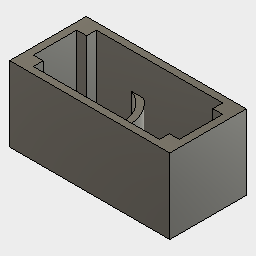
MG996R Body (Autodesk Fusion 360 design; units mm, degrees)
Autodesk Fusion 360 part; units mm, degrees
sketch "Base Sketch" plane through (0, 0, 0) normal (0, 1, 0) x (1, 0, 0)
  circle A0 centre (0, 0) radius 2.5 construction
  line L0 (-1.8028, 3) -> (1.8028, 3) construction
  line L1 (-1.8028, -3) -> (1.8028, -3) construction
  arc A1 (-1.8028, 3) -> (-1.8028, -3) centre (0, 0) ccw construction
  arc A2 (1.8028, -3) -> (1.8028, 3) centre (0, 0) ccw construction
  line L2 (-5, 5) -> (8, 5) construction
  line L3 (8, 5) -> (8, -5) construction
  line L4 (8, -5) -> (-5, -5) construction
  line L5 (-5, -5) -> (-5, 5) construction
  line L6 (8, 6) -> (-6, 6) construction
  line L7 (-6, 6) -> (-6, -6) construction
  line L8 (-6, -6) -> (8, -6) construction
  line L9 (8, -6) -> (8, 6) construction
  line L10 (8, 2.5) -> (6, 2.5) construction
  line L11 (6, 2.5) -> (6, 1.5) construction
  line L12 (6, 1.5) -> (8, 1.5) construction
  line L13 (8, 1.5) -> (8, 2.5) construction
  line L14 (8, -1.5) -> (6, -1.5) construction
  line L15 (6, -1.5) -> (6, -2.5) construction
  line L16 (6, -2.5) -> (8, -2.5) construction
  line L17 (8, -2.5) -> (8, -1.5) construction
  line L18 (-5, -6) -> (-1, -6) construction
  line L19 (-1, -6) -> (-1, -4) construction
  line L20 (-1, -4) -> (-5, -4) construction
  line L21 (-5, -4) -> (-5, -6) construction
  line L22 (2.5, 6) -> (6.5, 6) construction
  line L23 (6.5, 6) -> (6.5, 4) construction
  line L24 (6.5, 4) -> (2.5, 4) construction
  line L25 (2.5, 4) -> (2.5, 6) construction
  circle A3 centre (-20.5, 0) radius 8.5 construction
  circle A4 centre (-20.5, 0) radius 10 construction
  line L26 (8, 8) -> (-29, 8) construction
  line L27 (-29, 8) -> (-29, -8) construction
  line L28 (-29, -8) -> (8, -8) construction
  line L29 (8, -8) -> (8, 8) construction
  dimension "d1" = 5
  dimension "d2" = 7
  dimension "d3" = 6
  dimension "d4" = 3
  dimension "d5" = 10
  dimension "d6" = 5
  dimension "d7" = 5
  dimension "d8" = 13
  dimension "d9" = 1
  dimension "d10" = 1
  dimension "d11" = 1
  dimension "d12" = 2.5
  dimension "d13" = 2.5
  dimension "d14" = 1
  dimension "d15" = 2
  dimension "d16" = 4
  dimension "d17" = 2
  dimension "d18" = 4
  dimension "d19" = 2
  dimension "d20" = 7.5
  dimension "d21" = 17
  dimension "d22" = 1.5
  dimension "d23" = 4.5
  dimension "d24" = 37
  dimension "d25" = 16
  constraint coincident A0.centre A1.centre
  constraint horizontal L0
  constraint coincident A0.centre A1
  constraint parallel L0 L1
  constraint concentric A1 A2
  constraint horizontal L2
  constraint vertical L3
  constraint horizontal L4
  constraint vertical L5
  constraint horizontal L6
  constraint vertical L7
  constraint horizontal L8
  constraint vertical L9
  constraint collinear L3 L9
  constraint horizontal L10
  constraint vertical L11
  constraint horizontal L12
  constraint vertical L13
  constraint coincident L3 A0.centre
  constraint horizontal L14
  constraint vertical L15
  constraint horizontal L16
  constraint vertical L17
  constraint equal L10 L14
  constraint equal L11 L15
  constraint horizontal L18
  constraint vertical L19
  constraint horizontal L20
  constraint vertical L21
  constraint coincident L8 A0.centre
  constraint collinear L5 L21
  constraint horizontal L22
  constraint vertical L23
  constraint horizontal L24
  constraint vertical L25
  constraint coincident L6 A0.centre
  constraint horizontal A0.centre A1.centre
  constraint concentric A3 A4
  constraint coincident A4 A0.centre
  constraint horizontal L26
  constraint vertical L27
  constraint horizontal L28
  constraint vertical L29
  constraint collinear L3 L29
  constraint coincident L27 A0.centre
  constraint midpoint L27 A0.centre
  measures "d1" diameter of A0
  measures "d2" diameter of A1
  measures "d3" distance of L0 L1
  measures "d9" distance of L2 L6
  measures "d10" distance of L5 L7
  measures "d11" distance of L4 L8
  measures "d12" distance of L2 L10
  measures "d13" distance of L4 L16
  measures "d14" distance of A0.centre
  measures "d20" distance of L5 L25
  measures "d21" diameter of A3
  measures "d22" distance of A3 A4
sketch "Sketch2" plane through (0, 0, 0) normal (0, 1, 0) x (1, 0, 0)
  line L0 (8, 6) -> (-6, 6)
  line L1 (8, 5) -> (8, 6)
  line L2 (-6, 6) -> (-6, -6)
  line L3 (-6, -6) -> (8, -6)
  line L4 (8, -6) -> (8, -5)
  line L5 (8, -5) -> (-5, -5)
  line L6 (-5, -5) -> (-5, 5)
  line L7 (-5, 5) -> (8, 5)
extrude "Extrude1" add sketch "Sketch2" along normal blind 3.5 makes body 1
sketch "Sketch3" plane through (0, 3.5, 0) normal (0, 1, 0) x (-1, 0, 0)
  line L0 (5, -5) -> (-8, -5)
  line L1 (-8, -5) -> (-8, -6)
  line L2 (-8, -6) -> (6, -6)
  line L3 (6, -6) -> (6, 6)
  line L4 (6, 6) -> (-8, 6)
  line L5 (-8, 6) -> (-8, 5)
  line L6 (-8, 5) -> (5, 5)
  line L7 (5, 5) -> (5, -5)
  line L8 (-6.5, -5) -> (-2.5, -5)
  line L9 (-2.5, -5) -> (-2.5, -6)
  line L10 (-2.5, -6) -> (-6.5, -6)
  line L11 (-6.5, -6) -> (-6.5, -5)
  line L12 (-6.5, -6) -> (-6.5, -4)
  line L13 (5, 6) -> (1, 6)
  line L14 (1, 6) -> (1, 5)
  line L15 (1, 5) -> (5, 5)
  line L16 (5, 5) -> (5, 6)
  line L17 (1, 6) -> (1, 4)
  constraint horizontal L8
  constraint vertical L9
  constraint horizontal L10
  constraint vertical L11
  constraint midpoint origin L12
  constraint horizontal L13
  constraint vertical L14
  constraint horizontal L15
  constraint vertical L16
  constraint midpoint origin L17
extrude "Extrude2" add sketch "Sketch3" along normal blind 2.5 contours L0 L2 L8 L9 L10 L11 L12 | L4 L6 L13 L14 L15 L16 L17 bodies 1
sketch "Sketch4" plane through (0, 6, 0) normal (0, 1, 0) x (-1, 0, 0)
  line L0 (-2.5, -4) -> (-6.5, -4)
  line L1 (-6.5, -4) -> (-6.5, -6)
  line L2 (-6.5, -6) -> (-2.5, -6)
  line L3 (-2.5, -6) -> (-2.5, -4)
  line L4 (1, 4) -> (5, 4)
  line L5 (5, 4) -> (5, 6)
  line L6 (5, 6) -> (1, 6)
  line L7 (1, 6) -> (1, 4)
  constraint horizontal L0
  constraint vertical L1
  constraint horizontal L2
  constraint vertical L3
  constraint horizontal L4
  constraint vertical L5
  constraint horizontal L6
  constraint vertical L7
extrude "Extrude3" add sketch "Sketch4" along normal blind 1.5 bodies 1
sketch "Sketch5" plane through (0, 0, 0) normal (0, 1, 0) x (1, 0, 0)
  line L0 (8, 2.5) -> (6, 2.5)
  line L1 (6, 2.5) -> (6, 1.5)
  line L2 (6, 1.5) -> (8, 1.5)
  line L3 (8, 1.5) -> (8, 2.5)
  line L4 (6, -1.5) -> (8, -1.5)
  line L5 (8, -1.5) -> (8, -2.5)
  line L6 (8, -2.5) -> (6, -2.5)
  line L7 (6, -2.5) -> (6, -1.5)
  constraint horizontal L0
  constraint vertical L1
  constraint horizontal L2
  constraint vertical L3
  constraint horizontal L4
  constraint vertical L5
  constraint horizontal L6
  constraint vertical L7
extrude "Extrude4" add sketch "Sketch5" along normal blind 3.5 separate body makes body 2 at (6.6667, 2.3333, -2.5) makes body 3 at (6.6667, 2.3333, 2.5)
sketch "Sketch6" plane through (0, 0, 0) normal (0, 1, 0) x (1, 0, 0)
  circle A0 centre (0, 0) radius 2.5
  circle A1 centre (0, 0) radius 2.5
  arc A2 (1.8028, -3) -> (1.8028, 3) centre (0, 0) ccw
  line L0 (-1.8028, 3) -> (1.8028, 3)
  line L1 (-1.8028, -3) -> (1.8028, -3)
  arc A3 (1.8028, -3) -> (1.8028, 3) centre (0, 0) ccw
  arc A4 (-1.8028, 3) -> (-1.8028, -3) centre (0, 0) ccw
  constraint coincident A0.centre A1.centre
  constraint concentric A3 A4
extrude "Extrude5" add sketch "Sketch6" along normal blind 1 separate body makes body 4
sketch "Sketch7" plane through (0, 0, 0) normal (0, 1, 0) x (1, 0, 0)
  circle A0 centre (-20.5, 0) radius 8.5
  circle A1 centre (-20.5, 0) radius 8.5
  circle A2 centre (-20.5, 0) radius 10
  line L0 (-14.5, 8) -> (-17.6277, 8)
  line L1 (-14.5, -8) -> (-17.6277, -8)
  line L2 (-29, -8) -> (8, -8)
  line L3 (8, 8) -> (-29, 8)
  arc A3 (-17.6277, -8) -> (-17.6277, 8) centre (-20.5, 0) ccw
  arc A4 (-14.5, -8) -> (-14.5, 8) centre (-20.5, 0) ccw
  constraint coincident A2 origin
  constraint coincident A1 origin
  constraint parallel L0 L1
  constraint collinear L1 L2
  constraint collinear L0 L3
extrude "Extrude6" add sketch "Sketch7" along normal blind 10 separate body contours A0 A1 A2 L0 L1 L2 L3 A3 A4 makes body 5
sketch "Sketch8" plane through (0, 0, 0) normal (0, 1, 0) x (1, 0, 0)
  line L0 (-30.8, 9.7) -> (9.8, 9.7)
  line L1 (9.8, 9.7) -> (9.8, -9.7)
  line L2 (9.8, -9.7) -> (-30.8, -9.7)
  line L3 (-30.8, -9.7) -> (-30.8, 9.7)
  line L4 (8, -8) -> (8, 8)
  line L5 (-29, 8) -> (-29, -8)
  line L6 (8, 8) -> (-29, 8)
  line L7 (-29, -8) -> (8, -8)
  line L8 (-29, 8) -> (8, 8)
  line L9 (8, 8) -> (8, -8)
  line L10 (8, -8) -> (-29, -8)
  line L11 (-29, -8) -> (-29, 8)
  dimension "d38" = 1.8
  dimension "d39" = 1.8
  dimension "d40" = 1.7
  dimension "d41" = 1.7
  constraint horizontal L0
  constraint vertical L1
  constraint horizontal L2
  constraint vertical L3
  constraint horizontal L8
  constraint vertical L9
  constraint horizontal L10
  constraint vertical L11
  measures "d38" distance of L1 L4
  measures "d39" distance of L3 L5
  measures "d40" distance of L0 L6
  measures "d41" distance of L2 L7
extrude "Extrude7" add sketch "Sketch8" along normal blind 19 bodies 1 2 3 5
chamfer "Chamfer1" distance 1 angle 45 1 edges at (-3, 7.5, 4) on bodies 1
chamfer "Chamfer2" distance 1 angle 45 1 edges at (4.5, 7.5, -4) on bodies 1
sketch "Sketch9" plane through (0, 0, 0) normal (0, 1, 0) x (1, 0, 0)
  line L0 (-29, 8) -> (-26.5, 8)
  line L1 (-26.5, 8) -> (-26.5, 5.5)
  line L2 (-26.5, 5.5) -> (-29, 5.5)
  line L3 (-29, 5.5) -> (-29, 8)
  line L4 (-29, -8) -> (-26.5, -8)
  line L5 (-26.5, -8) -> (-26.5, -5.5)
  line L6 (-26.5, -5.5) -> (-29, -5.5)
  line L7 (-29, -5.5) -> (-29, -8)
  line L8 (8, 8) -> (5.5, 8)
  line L9 (5.5, 8) -> (5.5, 5.5)
  line L10 (5.5, 5.5) -> (8, 5.5)
  line L11 (8, 5.5) -> (8, 8)
  line L12 (8, -8) -> (5.5, -8)
  line L13 (5.5, -8) -> (5.5, -5.5)
  line L14 (5.5, -5.5) -> (8, -5.5)
  line L15 (8, -5.5) -> (8, -8)
  dimension "d46" = 2.5
  dimension "d47" = 2.5
  dimension "d48" = 2.5
  dimension "d49" = 2.5
  dimension "d50" = 2.5
  dimension "d51" = 2.5
  dimension "d52" = 2.5
  dimension "d53" = 2.5
  constraint horizontal L0
  constraint vertical L1
  constraint horizontal L2
  constraint vertical L3
  constraint horizontal L4
  constraint vertical L5
  constraint horizontal L6
  constraint vertical L7
  constraint horizontal L8
  constraint vertical L9
  constraint horizontal L10
  constraint vertical L11
  constraint horizontal L12
  constraint vertical L13
  constraint horizontal L14
  constraint vertical L15
extrude "Extrude8" add sketch "Sketch9" along normal blind 19 bodies 1
equation "d28 = 4 mm - 1.5 mm"
